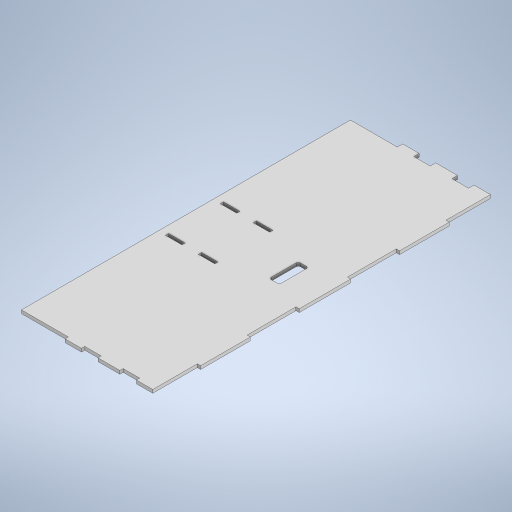
# Autodesk Inventor part: mieng_ben_gan_sensor_3mm
Saved by Autodesk Inventor 2023 (Build 270158000, 158)
## iProperties
Created: 2022-11-21
Part Number: mieng_ben_gan_sensor_3mm
Material: Generic
Document SubType Name: Modeling
Designer: ADMIN
Density: 1 g/cm^3
Appearance: Default
Author: ADMIN
Autodesk Inventor part; units mm, degrees
ref_plane "YZ Plane" through (0, 0, 0) normal (1, 0, 0) x (0, 1, 0)
ref_plane "XZ Plane" through (0, 0, 0) normal (0, 1, 0) x (-1, 0, 0)
ref_plane "XY Plane" through (0, 0, 0) normal (0, 0, 1) x (1, 0, 0)
sketch "Sketch1" plane through (0, 0, 0) normal (0, 1, 0) x (-1, 0, 0)
  line L0 (98.8824, -242.8336) -> (78.8824, -242.8336)
  line L1 (98.8824, -237.8336) -> (98.8824, -242.8336)
  line L2 (113.8824, -237.8336) -> (98.8824, -237.8336)
  line L3 (128.8824, -242.8336) -> (113.8824, -242.8336)
  line L4 (128.8824, -242.8336) -> (128.8824, -237.8336)
  line L5 (113.8824, -242.8336) -> (113.8824, -237.8336)
  line L6 (113.8824, 65.1664) -> (113.8824, 62.1664)
  line L7 (98.8824, 62.1664) -> (98.8824, 65.1664)
  line L8 (78.8824, 65.1664) -> (98.8824, 65.1664)
  line L9 (98.8824, 62.1664) -> (113.8824, 62.1664)
  line L10 (113.8824, 65.1664) -> (128.8824, 65.1664)
  line L11 (128.8824, 62.1664) -> (128.8824, 65.1664)
  line L12 (78.8824, 62.1664) -> (78.8824, 65.1664)
  line L13 (63.8824, 62.1664) -> (78.8824, 62.1664)
  line L14 (63.8824, 65.1664) -> (63.8824, 62.1664)
  line L15 (63.8824, -242.8336) -> (63.8824, -237.8336)
  line L16 (63.8824, -237.8336) -> (75.0605, -237.8336)
  line L17 (78.8824, -237.8336) -> (78.8824, -242.8336)
  line L18 (78.8824, -237.8336) -> (63.8824, -237.8336)
  line L19 (63.8824, -237.8336) -> (78.8824, -237.8336)
  line L20 (48.8824, -65.4156) -> (48.8824, -20.7764)
  line L21 (48.8824, -65.4156) -> (48.8824, -20.7764)
  line L22 (48.8824, -65.4156) -> (45.8824, -65.4156)
  line L23 (45.8824, -112.2516) -> (45.8824, -65.4156)
  line L24 (48.8824, -20.7764) -> (45.8824, -20.7764)
  line L25 (48.8824, -202.2369) -> (45.8824, -202.2369)
  line L26 (48.8824, -156.8908) -> (45.8824, -156.8908)
  line L27 (45.8824, -202.2369) -> (45.8824, -156.8908)
  line L28 (48.8824, -112.2516) -> (45.8824, -112.2516)
  line L29 (48.8824, -156.8908) -> (48.8824, -112.2516)
  line L30 (48.8824, -156.8908) -> (48.8824, -112.2516)
  line L31 (45.8824, -20.7764) -> (45.8824, 24.5697)
  line L32 (48.8824, 24.5697) -> (45.8824, 24.5697)
  line L33 (48.8824, 24.5697) -> (48.8824, 62.1664)
  line L34 (48.8824, 65.1664) -> (63.8824, 65.1664)
  line L35 (48.8824, 24.5697) -> (48.8824, 65.1664)
  line L36 (48.8824, -237.8336) -> (48.8824, -202.2369)
  line L37 (48.8824, -242.8336) -> (63.8824, -242.8336)
  line L38 (48.8824, -242.8336) -> (48.8824, -237.8336)
  line L39 (164.8824, -115.3336) -> (164.8824, -112.3336)
  line L40 (164.8824, -112.3336) -> (149.8824, -112.3336)
  line L41 (149.8824, -112.3336) -> (149.8824, -115.3336)
  line L42 (134.8824, -115.3336) -> (134.8824, -112.3336)
  line L43 (134.8824, -112.3336) -> (119.8824, -112.3336)
  line L44 (119.8824, -112.3336) -> (119.8824, -115.3336)
  line L45 (119.8824, -115.3336) -> (134.8824, -115.3336)
  line L46 (149.8824, -115.3336) -> (164.8824, -115.3336)
  line L47 (171.6524, -88.8336) -> (171.6524, -237.8336)
  line L48 (171.6524, -237.8336) -> (128.8824, -237.8336)
  line L49 (171.6524, -88.8336) -> (171.6524, 62.1664)
  line L50 (171.6524, 62.1664) -> (128.8824, 62.1664)
  line L51 (164.8824, -62.3336) -> (164.8824, -65.3336)
  line L52 (164.8824, -65.3336) -> (149.8824, -65.3336)
  line L53 (149.8824, -65.3336) -> (149.8824, -62.3336)
  line L54 (134.8824, -62.3336) -> (134.8824, -65.3336)
  line L55 (134.8824, -65.3336) -> (119.8824, -65.3336)
  line L56 (119.8824, -65.3336) -> (119.8824, -62.3336)
  line L57 (119.8824, -62.3336) -> (134.8824, -62.3336)
  line L58 (149.8824, -62.3336) -> (164.8824, -62.3336)
  line L59 (76.2158, -102.1043) -> (81.5491, -102.1043)
  line L60 (83.5491, -100.1043) -> (83.5491, -77.5629)
  line L61 (81.5491, -75.5629) -> (76.2158, -75.5629)
  line L62 (74.2158, -77.5629) -> (74.2158, -100.1043)
  line L63 (74.2158, -102.1043) -> (83.5491, -75.5629) construction
  line L64 (83.5491, -102.1043) -> (74.2158, -75.5629) construction
  arc A0 (83.5491, -77.5629) -> (81.5491, -75.5629) centre (81.5491, -77.5629) ccw
  arc A1 (76.2158, -75.5629) -> (74.2158, -77.5629) centre (76.2158, -77.5629) ccw
  arc A2 (81.5491, -102.1043) -> (83.5491, -100.1043) centre (81.5491, -100.1043) ccw
  arc A3 (74.2158, -100.1043) -> (76.2158, -102.1043) centre (76.2158, -100.1043) ccw
  point P0 (0, 0)
  point P1 (0, 0)
  point P2 (106.3824, -237.8336)
  point P3 (106.3824, 62.1664)
  point P4 (121.3824, 65.1664)
  point P5 (47.3824, -202.2369)
  point P6 (78.8824, -88.8336)
  dimension "d0" = 80
  dimension "d1" = 15
  dimension "d2" = 15
  dimension "d3" = 300
  dimension "d5" = 3
  dimension "d6" = 5
  dimension "d7" = 44.6392
  dimension "d8" = 37.5967
  dimension "d9" = 44.6392
  dimension "d10" = 40.5967
  dimension "d11" = 45.3461
  dimension "d12" = 46.8359
  dimension "d13" = 45.3461
  dimension "d14" = 20
  dimension "d15" = 15
  dimension "d16" = 15
  dimension "d17" = 15
  dimension "d18" = 15
  dimension "d19" = 15
  dimension "d20" = 15
  dimension "d21" = 20
  dimension "d22" = 308
  dimension "d29" = 3
  dimension "d30" = 15
  dimension "d31" = 3
  dimension "d32" = 15
  dimension "d33" = 3
  dimension "d34" = 15
  dimension "d38" = 2
  constraints: 130 end point, 21 perpendicular, 14 point on line, 8 parallel, 8 point on circle, 8 tangent, 6 horizontal, 6 midpoint, 4 centre point, 3 equal radius, 2 vertical
  measures "d0" distance of L4.end L36.start
  measures "d1" distance of L38.start L37.end
  measures "d2" distance of L16.start L19.end
  measures "d3" distance of point (106.382, -237.834) point (106.382, 62.166)
  measures "d5" vertical distance of L6.end point (121.382, 65.166)
  measures "d6" distance between parallel lines of L2 L3
  measures "d7" distance of L22.start L24.start
  measures "d8" distance of L32.start L33.end
  measures "d9" distance of L26.start L29.end
  measures "d10" distance from line of L37 point (47.382, -202.237)
  measures "d11" distance of L25.end L26.end
  measures "d12" distance of L28.end L23.end
  measures "d13" distance of L24.end L31.end
  measures "d14" distance of L12.end L8.end
  measures "d15" distance of L7.start L6.end
  measures "d16" distance of L6.start L11.end
  measures "d17" distance of L35.end L34.end
  measures "d18" distance of L13.start L13.end
  measures "d19" distance of L3.start L3.end
  measures "d20" distance of L2.start L2.end
  measures "d21" distance of L1.end L0.end
  measures "d22" distance between parallel lines of L3 L10
  measures "d29" distance of L39.start L39.end
  measures "d30" distance of L39.end L40.end
  measures "d31" distance of L40.end L41.end
  measures "d32" distance of L41.end L42.start
  measures "d33" distance of L42.start L42.end
  measures "d34" distance of L42.end L43.end
  measures "d38" radius of A0
extrude "Extrusion1" add sketch "Sketch1" along normal blind 3
body "Solid1"
